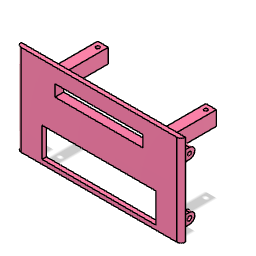
Panneau frontal avec support CàP (Autodesk Fusion 360 design; units mm, degrees)
Autodesk Fusion 360 part; units mm, degrees
sketch "Sketch1" plane through (0, 0, 0) normal (0, -1, 0) x (1, 0, 0)
  line L0 (68.9136, 128.1911) -> (-39.0864, 128.1911)
  line L1 (-39.0864, 128.1911) -> (-39.0864, -30.8089)
  line L2 (-39.0864, -30.8089) -> (68.9136, -30.8089)
  line L3 (68.9136, -30.8089) -> (68.9136, 128.1911)
  line L4 (-42.0864, 131.1911) -> (71.9136, 131.1911)
  line L5 (71.9136, 131.1911) -> (71.9136, 128.1911)
  line L6 (71.9136, 128.1911) -> (-42.0864, 128.1911)
  line L7 (-42.0864, 128.1911) -> (-42.0864, 131.1911)
  dimension "d35_1" = 114
  dimension "d36_1" = 3
  dimension "d37_1" = 3
  constraint horizontal L4
  constraint vertical L5
  constraint horizontal L6
  constraint vertical L7
  constraint collinear L0 L6
  measures "d35_1" distance of L4.start L4.end
  measures "d36_1" distance of L4.start L6.end
  measures "d37_1" distance of L1 L7
extrude "Extrude Façade" add sketch "Sketch1" against normal blind 63 contours L0 L4 L5 L6 L7 makes body 1
sketch "Sketch2" plane through (0, 0, 131.1911) normal (0, 0, 1) x (1, 0, 0)
  line L0 (-42.0864, 0) -> (71.9136, 0)
  line L1 (71.9136, 0) -> (71.9136, 63)
  line L2 (71.9136, 63) -> (-42.0864, 63)
  line L3 (-42.0864, 63) -> (-42.0864, 0)
  line L4 (-12.5864, 49.9) -> (42.4136, 49.9)
  line L5 (42.4136, 49.9) -> (42.4136, 47.9)
  line L6 (42.4136, 47.9) -> (-12.5864, 47.9)
  line L7 (-12.5864, 47.9) -> (-12.5864, 49.9)
  point P0 (14.9136, 0)
  dimension "d41_1" = 55
  dimension "d42_1" = 2
  dimension "d43_1" = 49.9
  dimension "d44_1" = 27.5
  constraint horizontal L4
  constraint vertical L5
  constraint horizontal L6
  constraint vertical L7
  constraint midpoint L0 P0
  measures "d41_1" distance of L4.start L4.end
  measures "d42_1" distance of L4.start L6.end
  measures "d43_1" distance of L0 L4
  measures "d44_1" distance of L7 P0
extrude "Extrude fente CàP" cut sketch "Sketch2" against normal blind 3 contours L4 L5 L6 L7 bodies 1
chamfer "Chanfrein Fente CàP" distance 3 angle 45 4 edges at (14.9136, 49.9, 131.1911) (-12.5864, 48.9, 131.1911) (14.9136, 47.9, 131.1911) (42.4136, 48.9, 131.1911) on bodies 1
ref_plane "WorkPlane1" through (68.4136, 31.5, 129.6911) normal (1, 0, 0) x (0, 0, -1)
sketch "Sketch5" plane through (68.4136, 31.5, 129.6911) normal (1, 0, 0) x (0, 0, -1)
  circle A0 centre (7.85, 16.85) radius 1.25
  circle A1 centre (7.85, 16.85) radius 3.65
  line L0 (1.5, -31.5) -> (1.5, 31.5) construction
  line L1 (11.5, 18.4087) -> (11.5, 13.1241) construction
  line L2 (4.6605, 20.5) -> (14.2431, 20.5) construction
  line L3 (-1.5, -31.5) -> (1.5, -31.5) construction
  line L4 (1.5, 20.5) -> (9.6841, 20.5)
  line L5 (1.5, 13.2) -> (8.9714, 13.2)
  line L6 (1.5, 20.5) -> (1.5, 13.2)
  dimension "d52_1" = 2.5
  dimension "d53_1" = 2.4
  dimension "d55_1" = 10
  dimension "d56_1" = 52
  constraint vertical L1
  constraint tangent A1 L1
  constraint horizontal L2
  constraint tangent A1 L2
  constraint coincident L0 L4.start
  constraint perpendicular L0 L4
  constraint coincident L0 L5.start
  constraint perpendicular L0 L5
  constraint tangent A1 L4
  constraint tangent A1 L5
  measures "d52_1" diameter of A0
  measures "d55_1" distance of L0 L1
  measures "d56_1" distance of L2 L3
extrude "Extrude Fixations supérieures" add sketch "Sketch5" against normal blind 9 bodies 1
fillet "Fillet Fixations supérieures" radius 2 3 edges at (63.9136, 52, 128.1911) (59.4136, 48.35, 128.1911) (63.9136, 44.7, 128.1911) on bodies 1
copy_body "CopyPasteBodies1" bodies 1 makes body 2
sketch "Sketch6" plane through (68.4136, 31.5, 129.6911) normal (1, 0, 0) x (0, 0, -1)
  line L0 (11.5, -18.8864) -> (11.5, -29.6025) construction
  line L1 (1.5, -31.5) -> (1.5, 31.5) construction
  circle A0 centre (7.85, -22.15) radius 1.5
  circle A1 centre (7.85, -22.15) radius 3.65
  line L2 (1.5, -28.5) -> (160.5, -28.5)
  line L3 (1.5, -18.5) -> (9.3221, -18.5)
  line L4 (11.5, -24.3654) -> (11.5, -28.5)
  line L5 (1.5, -18.5) -> (1.5, -28.5)
  line L6 (1.5, -25.8) -> (9.9241, -25.8)
  dimension "d63_1" = 10
  dimension "d64_1" = 3
  dimension "d65_1" = 2.15
  dimension "d213_1" = 10
  constraint vertical L0
  constraint tangent L0 A1
  constraint coincident L1 L3.start
  constraint perpendicular L1 L3
  constraint coincident L2.start L5.end
  constraint tangent A1 L3
  constraint coincident L2 L4.end
  constraint perpendicular L2 L4
  constraint tangent A1 L4
  constraint coincident L5 L6.start
  constraint perpendicular L5 L6
  constraint tangent A1 L6
  measures "d63_1" distance of L0 L1
  measures "d64_1" diameter of A0
  measures "d213_1" distance of L2 L3
extrude "Extrude fixation inférieures" add sketch "Sketch6" against normal blind 3 bodies 1 2
fillet "Fillet2" radius 2 3 edges at (66.9136, 13, 128.1911) (66.9136, 5.7, 128.1911) (65.4136, 9.35, 128.1911) on bodies 1
ref_plane "WorkPlane2" through (14.9136, 31.5, 129.6911) normal (1, 0, 0) x (0, 0, -1)
mirror "Mirror2" about plane through (14.9136, 31.5, 129.6911) normal (1, 0, 0) of "Extrude Fixations supérieures", "Fillet Fixations supérieures", "Extrude fixation inférieures", "Fillet2"
ref_plane "WorkPlane3" through (14.9136, 31.5, 129.6911) normal (1, 0, 0) x (0, 0, -1)
ref_plane "WorkPlane4" through (56.0636, 31.5, 129.6911) normal (1, 0, 0) x (0, 0, -1)
sketch "Sketch8" plane through (56.0636, 31.5, 129.6911) normal (1, 0, 0) x (0, 0, -1)
  line L0 (1.5, 21.5) -> (38.8, 21.5)
  line L1 (1.5, -31.5) -> (1.5, 31.5)
  line L2 (1.5, 21.5) -> (38.8, 21.5)
  line L3 (38.8, 21.5) -> (38.8, 11.5)
  line L4 (38.8, 11.5) -> (1.5, 11.5)
  line L5 (1.5, 11.5) -> (1.5, 21.5)
  point P0 (1.5, -31.5)
  dimension "d223" = 53
  dimension "d224" = 37.3
  dimension "d225" = 10
  constraint horizontal L0
  constraint coincident L0.start L1
  constraint horizontal L2
  constraint vertical L3
  constraint horizontal L4
  constraint vertical L5
  constraint coincident L0.end L3
  measures "d223" distance of L0 P0
  measures "d224" distance of L0.start L0.end
  measures "d225" distance of L0.start L4.end
extrude "Extrude7" add sketch "Sketch8" against normal blind 7.3 bodies 1
sketch "Sketch9" plane through (0, 53, 0) normal (0, 1, 0) x (-1, 0, 0)
  line L0 (-56.0636, 128.1911) -> (-56.0636, 90.8911)
  line L1 (-56.0636, 90.8911) -> (-48.7636, 90.8911)
  line L2 (-48.7636, 90.8911) -> (-48.7636, 128.1911)
  line L3 (-48.7636, 128.1911) -> (-56.0636, 128.1911)
  circle A0 centre (-52.4136, 120.6411) radius 1.25
  line L4 (-52.4136, 128.1911) -> (-52.4136, 116.6122) construction
  circle A1 centre (-52.4136, 94.5411) radius 1.25
  point P0 (-52.4136, 128.1911)
  dimension "d228" = 2.5
  dimension "d229" = 7.55
  dimension "d232" = 2.5
  dimension "d233" = 26.1
  constraint midpoint L3 P0
  constraint coincident P0 L4.start
  constraint perpendicular L3 L4
  constraint coincident A0.centre L4
  constraint coincident L4 A1.centre
  measures "d228" diameter of A0
  measures "d229" vertical distance of L2.end A0.centre
  measures "d232" diameter of A1
  measures "d233" vertical distance of A0.centre A1.centre
extrude "Extrude8" cut sketch "Sketch9" against normal blind 10 contours A0 | A1 bodies 1
fillet "Fillet3" radius 2 4 edges at (52.4136, 53, 128.1911) (56.0636, 48, 128.1911) (52.4136, 43, 128.1911) (48.7636, 48, 128.1911) on bodies 1
mirror "Mirror3" about plane through (14.9136, 31.5, 129.6911) normal (1, 0, 0) of "Extrude7", "Extrude8", "Fillet3"
fillet "Fillet5" radius 3 4 edges at (-42.0864, 31.5, 131.1911) (-42.0864, 31.5, 131.1911) (71.9136, 31.5, 131.1911) (71.9136, 31.5, 131.1911) on bodies 1 2
sketch "Ouverture tiroir" plane through (0, 0, 131.1911) normal (0, 0, 1) x (1, 0, 0)
  line L0 (68.9136, 0) -> (68.9136, 63)
  line L1 (68.9136, 63) -> (-39.0864, 63)
  line L2 (-39.0864, 63) -> (-39.0864, 0)
  line L3 (-39.0864, 0) -> (68.9136, 0)
  line L4 (45.4136, 52.9) -> (45.4136, 44.9)
  line L5 (45.4136, 44.9) -> (-15.5864, 44.9)
  line L6 (-15.5864, 44.9) -> (-15.5864, 52.9)
  line L7 (-15.5864, 52.9) -> (45.4136, 52.9)
  line L8 (-24.5864, 23.5) -> (54.4136, 23.5)
  line L9 (54.4136, 23.5) -> (54.4136, 3)
  line L10 (54.4136, 3) -> (-24.5864, 3)
  line L11 (-24.5864, 3) -> (-24.5864, 23.5)
  line L12 (71.9136, 0) -> (71.9136, 63)
  dimension "d340" = 79
  dimension "d341" = 20.5
  dimension "d343" = 17.5
  dimension "d344" = 3
  constraint horizontal L8
  constraint vertical L9
  constraint horizontal L10
  constraint vertical L11
  measures "d340" distance of L8.start L8.end
  measures "d341" distance of L8.start L10.end
  measures "d343" distance of L9 L12
  measures "d344" distance of L3 L10
extrude "Extrude10" cut sketch "Ouverture tiroir" against normal blind 3 contours L8 L9 L10 L11 bodies 1
equation "d35_1 = Largeur + 2 * EpaisseurParoi"
equation "d36_1 = EpaisseurParoi"
equation "d37_1 = EpaisseurParoi"
equation "d39_1 = -HauteurPanneauFrontal"
equation "d43_1 = HauteurPlatineCàP + EpaisseurParoi - 3.6 mm + Tolerance"
equation "d44_1 = ( 55 / 2 ) * 1 mm"
equation "d45_1 = -EpaisseurParoi"
equation "d47_1 = EpaisseurParoi"
equation "d51_1 = -EpaisseurParoi - Tolerance"
equation "d52_1 = PerçageO3"
equation "d53_1 = EpaisseurParoiPerçage"
equation "d56_1 = HauteurPlatineCàP + EpaisseurParoi - 2 * Tolerance"
equation "d222 = ( 75 / 2 ) * 1 mm + 3.65 mm"
equation "d223 = EpaisseurParoi + HauteurPlatineCàP"
equation "d224 = 7.05 mm + Tolerance + 26.1 mm + 3.65 mm"
equation "d228 = PerçageO3"
equation "d229 = 7.05 mm + Tolerance"
equation "d232 = PerçageO3"
equation "d275 = EpaisseurParoi"
equation "d340 = LargeurTiroir + 2 * Tolerance"
equation "d341 = Hauteurtiroir + Tolerance"
equation "d343 = ( Largeur + 2 * EpaisseurParoi - LargeurTiroir ) / 2 - Tolerance"
equation "d344 = EpaisseurParoi"
equation "d345 = -EpaisseurParoi"
equation "Largeur = 108 mm"
equation "EpaisseurParoi = 3 mm"
equation "Tolerance = 0.5 mm"
equation "PerçageO3 = 2.5 mm"
equation "EpaisseurParoiPerçage = 2.4 mm"
equation "HauteurPlatineCàP = 50 mm"
equation "HauteurPanneauFrontal = HauteurPlatineCàP + 10 mm + EpaisseurParoi"
equation "LargeurTiroir = 78 mm"
equation "Hauteurtiroir = 20 mm"
